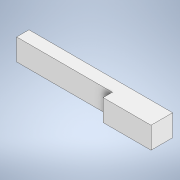
# Autodesk Inventor part: Key--E
Saved by Autodesk Inventor 2021 (Build 250183000, 183)
## iProperties
Created: 2021-03-17
Part Number: Key--E
Material: Generic
Document SubType Name: Modeling
Designer: Tom
Density: 1 g/cm^3
Appearance: White
Author: Tom
Autodesk Inventor part; units mm, degrees
ref_plane "YZ Plane" through (0, 0, 0) normal (1, 0, 0) x (0, 1, 0)
ref_plane "XZ Plane" through (0, 0, 0) normal (0, 1, 0) x (-1, 0, 0)
ref_plane "XY Plane" through (0, 0, 0) normal (0, 0, 1) x (1, 0, 0)
sketch "Sketch1" plane through (0, 0, 0) normal (0, 1, 0) x (-1, 0, 0)
  line L0 (0, 0) -> (147.6375, 0)
  line L1 (147.6375, 0) -> (147.6375, 12.7)
  line L2 (147.6375, 12.7) -> (49.2125, 12.7)
  line L3 (49.2125, 12.7) -> (49.2125, 22.225)
  line L4 (49.2125, 22.225) -> (0, 22.225)
  line L5 (0, 22.225) -> (0, 0)
  dimension "d0" = 147.6375
  dimension "d1" = 98.425
  dimension "d2" = 22.225
  dimension "d3" = 12.7
  constraints: 12 end point, 5 perpendicular, 1 horizontal
  measures "d0" distance of L0.start L0.end
  measures "d1" distance of L1.end L2.end
  measures "d2" distance of L4.end L0.start
  measures "d3" distance between parallel lines of L2 L0
extrude "Extrusion1" add sketch "Sketch1" against normal blind 22.225
body "Solid1"
